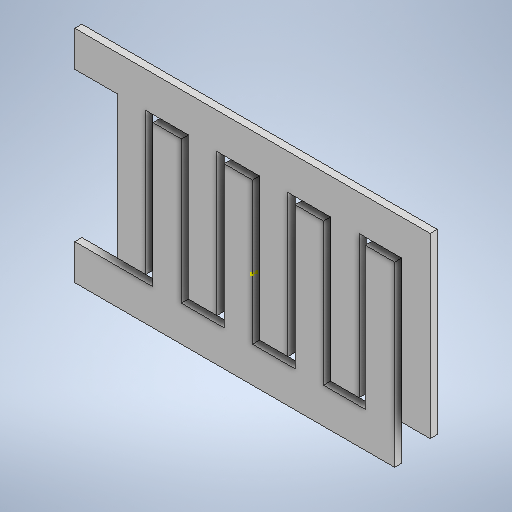
# Autodesk Inventor part: Part4
Saved by Autodesk Inventor 2025.2 (Build 292293000, 293)
## iProperties
Created: 2025-01-26
Part Number: Part4
Material: Generic
Document SubType Name: Modeling
Designer: ishad
Density: 1 g/cm^3
Appearance: Default
Author: ishad
## iProperties of the stored document Sensor-001-001_3DPrint.ipt
Created: 2025-01-26
Part Number: Sensor-001-001_3DPrint
Material: Generic
Document SubType Name: Modeling
Designer: ishad
Density: 1 g/cm^3
Appearance: Default
Author: ishad
Autodesk Inventor part; units mm, degrees
ref_plane "YZ Plane" through (0, 0, 0) normal (1, 0, 0) x (0, 1, 0)
ref_plane "XZ Plane" through (0, 0, 0) normal (0, 1, 0) x (-1, 0, 0)
ref_plane "XY Plane" through (0, 0, 0) normal (0, 0, 1) x (1, 0, 0)
sketch "Sketch1" plane through (0, 0, 0) normal (0, 0, 1) x (1, 0, 0)
  point P0 (0, 0)
sketch "Sketch2" plane through (0, 0, 0) normal (0, 0, 1) x (1, 0, 0)
  line L0 (-25, 17.5) -> (25, 17.5)
  line L1 (25, 17.5) -> (25, -7.5)
  line L2 (-25, 17.5) -> (-20, 17.5)
  line L3 (-25, 17.5) -> (-25, 12.5)
  line L4 (25, -7.5) -> (21, -7.5)
  line L5 (21, -7.5) -> (21, 12.5)
  line L6 (21, 12.5) -> (15, 12.5)
  line L7 (15, 12.5) -> (15, -7.5)
  line L8 (15, -7.5) -> (11, -7.5)
  line L9 (11, -7.5) -> (11, 12.5)
  line L10 (11, 12.5) -> (5, 12.5)
  line L11 (5, 12.5) -> (5, -7.5)
  line L12 (5, -7.5) -> (1, -7.5)
  line L13 (1, -7.5) -> (1, 12.5)
  line L14 (1, 12.5) -> (-5, 12.5)
  line L15 (-5, 12.5) -> (-5, -7.5)
  line L16 (-5, -7.5) -> (-9, -7.5)
  line L17 (-9, -7.5) -> (-9, 12.5)
  line L18 (-9, 12.5) -> (-15, 12.5)
  line L19 (-15, 12.5) -> (-15, -7.5)
  line L20 (-15, -7.5) -> (-19, -7.5)
  line L21 (-19, -7.5) -> (-19, 12.5)
  line L22 (-25, 12.5) -> (-19, 12.5)
  line L23 (20, 11.5) -> (15.875, 11.5)
  line L24 (15.875, 11.5) -> (15.875, -7.5)
  line L25 (15.875, -7.5) -> (15.875, -8.5)
  line L26 (15.875, -8.5) -> (10, -8.5)
  line L27 (10, -8.5) -> (10, 11.5)
  line L28 (10, 11.5) -> (6, 11.5)
  line L29 (6, 11.5) -> (6, -8.5)
  line L30 (6, -8.5) -> (0, -8.5)
  line L31 (0, -8.5) -> (0, 11.5)
  line L32 (0, 11.5) -> (-4, 11.5)
  line L33 (-4, 11.5) -> (-4, -8.5)
  line L34 (-4, -8.5) -> (-10, -8.5)
  line L35 (-10, -8.5) -> (-10, 3.175)
  line L36 (-10, 11.5) -> (-10, 3.175)
  line L37 (-10, 11.5) -> (-14, 11.5)
  line L38 (-14, 11.5) -> (-14, 3.175)
  line L39 (-14, -8.5) -> (-14, 3.175)
  line L40 (-14, -8.5) -> (-25, -8.5)
  line L41 (-25, -13.5) -> (20, -13.5)
  line L42 (20, 11.5) -> (20, -13.5)
  line L43 (-25, -8.5) -> (-25, -13.5)
  point P0 (0, 0)
  dimension "d8" = 50
  dimension "d11" = 5
  dimension "d13" = 4
  dimension "d14" = 25
  dimension "d16" = 6
  dimension "d27" = 6
  dimension "d28" = 6
  dimension "d29" = 6
  dimension "d30" = 6
  dimension "d48" = 5
  constraints: 88 end point, 15 perpendicular, 11 horizontal, 11 point on line, 10 vertical, 3 parallel, 1 collinear
  measures "d8" distance of L0.start L0.end
  measures "d11" distance of L0.start L3.end
  measures "d13" distance of L1.end L4.end
  measures "d14" distance of L0.end L1.end
  measures "d16" distance of L5.end L6.end
  measures "d27" distance of L17.end L18.end
  measures "d28" distance of L13.end L14.end
  measures "d29" distance of L9.end L10.end
  measures "d30" distance of L3.end L21.end
  measures "d48" distance of L40.end L41.start
sketch "Sketch3" plane through (0, 0, 0) normal (0, 0, 1) x (1, 0, 0)
  point P0 (0, 0)
extrude "Extrusion1" add sketch "Sketch2" along normal mid plane 1
sketch "Sketch4" plane through (0, 0, 0.5) normal (0, 0, 1) x (1, 0, 0)
  point P0 (0, 0)
body "Solid1"
